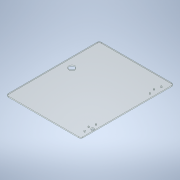
# Autodesk Inventor part: Puerta Lateral Derecha
Saved by Autodesk Inventor 2020 (Build 240168000, 168)
## iProperties
Created: 2020-06-12
Part Number: Puerta Lateral Derecha
Material: Genérico
Document SubType Name: Modeling
Designer: Pipi
Density: 1 g/cm^3
Appearance: Claro
Author: Pipi
Autodesk Inventor part; units mm, degrees
ref_plane "YZ Plane" through (0, 0, 0) normal (1, 0, 0) x (0, 1, 0)
ref_plane "XZ Plane" through (0, 0, 0) normal (0, 1, 0) x (-1, 0, 0)
ref_plane "XY Plane" through (0, 0, 0) normal (0, 0, 1) x (1, 0, 0)
sketch "Boceto1" plane through (0, 0, 0) normal (0, 1, 0) x (-1, 0, 0)
  line L0 (64.9389, -223.5898) -> (-165.0611, -223.5898)
  line L1 (-172.0611, -216.5898) -> (-172.0611, 73.4102)
  line L2 (-165.0611, 80.4102) -> (64.9389, 80.4102)
  line L3 (71.9389, 73.4102) -> (71.9389, -216.5898)
  circle A0 centre (-157.4361, -196.7148) radius 2
  circle A1 centre (-157.4361, -159.4648) radius 2
  circle A2 centre (-152.2061, -178.0898) radius 2
  circle A3 centre (-157.4361, 53.5352) radius 2
  circle A4 centre (-157.4361, 16.2852) radius 2
  circle A5 centre (-152.2061, 34.9102) radius 2
  circle A6 centre (-165.0611, 34.9102) radius 4
  circle A7 centre (41.9389, -104.5898) radius 9.5
  arc A8 (64.9389, -223.5898) -> (71.9389, -216.5898) centre (64.9389, -216.5898) ccw
  arc A9 (-172.0611, -216.5898) -> (-165.0611, -223.5898) centre (-165.0611, -216.5898) ccw
  arc A10 (-165.0611, 80.4102) -> (-172.0611, 73.4102) centre (-165.0611, 73.4102) ccw
  arc A11 (71.9389, 73.4102) -> (64.9389, 80.4102) centre (64.9389, 73.4102) ccw
  point P0 (0, 0)
  point P1 (63.9389, -223.5898)
  point P2 (71.9389, -215.5898)
  point P3 (-172.0611, -215.5898)
  point P4 (-164.0611, -223.5898)
  point P5 (-172.0611, 72.4102)
  point P6 (-164.0611, 80.4102)
  point P7 (63.9389, 80.4102)
  point P8 (71.9389, 72.4102)
  dimension "d10" = 4
  dimension "d11" = 14.625
  dimension "d12" = 26.875
  dimension "d13" = 4
  dimension "d14" = 37.25
  dimension "d15" = 14.625
  dimension "d16" = 4
  dimension "d17" = 18.625
  dimension "d18" = 19.855
  dimension "d19" = 8
  dimension "d20" = 7
  dimension "d21" = 19
  dimension "d22" = 30
  dimension "d23" = 244
  dimension "d24" = 304
  dimension "d25" = 7
  dimension "d26" = 7
  dimension "d27" = 7
  dimension "d28" = 185
  constraints: 12 centre point, 8 end point, 8 point on circle, 8 point on line, 8 tangent, 2 parallel, 1 equal radius, 1 horizontal, 1 perpendicular
  measures "d10" diameter of A0
  measures "d11" distance from line of L1 A0.centre
  measures "d12" distance from line of L0 A0.centre
  measures "d13" diameter of A1
  measures "d14" distance of A0.centre A1.centre
  measures "d15" distance from line of L1 A1.centre
  measures "d16" diameter of A2
  measures "d17" vertical distance of A2.centre A1.centre
  measures "d18" distance from line of L1 A2.centre
  measures "d19" diameter of A6
  measures "d20" distance from line of L1 A6.centre
  measures "d21" diameter of A7
  measures "d22" distance from line of L3 A7.centre
  measures "d23" distance between parallel lines of L3 L1
  measures "d24" distance between parallel lines of L2 L0
  measures "d25" radius of A8
  measures "d26" radius of A9
  measures "d27" radius of A10
  measures "d28" distance from line of L2 A7.centre
extrude "Extrusión1" add sketch "Boceto1" along normal blind 3
